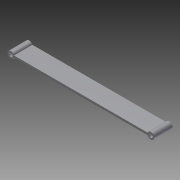
# Autodesk Inventor part: x-IMU Calibration Cube Bracket0
Saved by Autodesk Inventor 2011 (Build 150239000, 239)
## iProperties
Created: 2012-03-21
Part Number: x-IMU Calibration Cube Bracket0
Document SubType Name: Modeling
Designer: Seb Madgwick
Density: 1 g/cm^3
Author: Seb Madgwick
Autodesk Inventor part; units mm, degrees
ref_plane "YZ Plane" through (0, 0, 0) normal (1, 0, 0) x (0, 1, 0)
ref_plane "XZ Plane" through (0, 0, 0) normal (0, 1, 0) x (-1, 0, 0)
ref_plane "XY Plane" through (0, 0, 0) normal (0, 0, 1) x (1, 0, 0)
sketch "Sketch1" plane through (0, 0, 0) normal (0, 0, 1) x (1, 0, 0)
  line L0 (0, 1.5) -> (0, -1.5)
  line L1 (0, 1.5) -> (-90.7044, 1.5)
  line L2 (-90.7044, -1.5) -> (0, -1.5)
  arc A0 (-90.7044, 1.5) -> (-90.7044, -1.5) centre (-95, 0) ccw
  circle A1 centre (-95, 0) radius 2.5
  point P0 (0, 0)
  dimension "d4" = 95
  dimension "d6" = 5
  dimension "d8" = 2.05
  dimension "d12" = 3
  dimension "d13" = 0
  dimension "d14" = 1.5
  constraints: 6 end point, 2 centre point, 2 point on circle, 1 coincident, 1 parallel, 1 perpendicular, 1 vertical
  measures "d4" distance from line of L0 A0.centre
  measures "d6" diameter of A1
  measures "d8" radial gap between concentric circles of A0 A1
  measures "d12" distance between parallel lines of L2 L1
  measures "d13" distance from line of L0 point (0, 0)
  measures "d14" distance from line of L2 point (0, 0)
extrude "Extrusion1" add sketch "Sketch1" along normal mid plane 25
mirror "Mirror1" about plane through (0, 0, 0) normal (1, 0, 0) of "Extrusion1"
equation "\"d14\" = 0.5 * d12"
body "Solid1"
